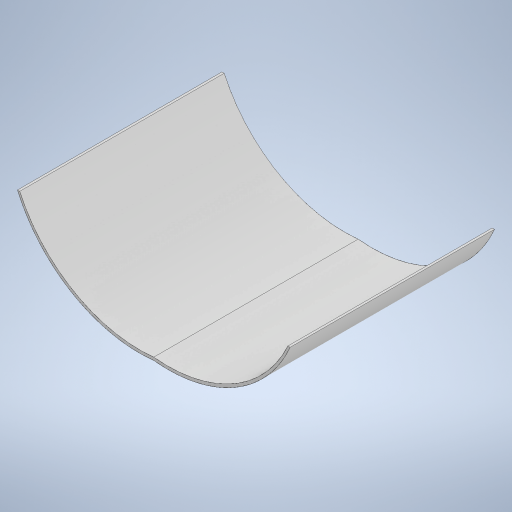
# Autodesk Inventor part: Base
Saved by Autodesk Inventor 2024 (Build 280153000, 153)
## iProperties
Created: 2024-09-04
Part Number: Base
Material: Generic
Document SubType Name: Modeling
Designer: srira
Density: 1 g/cm^3
Appearance: Default
Author: srira
Autodesk Inventor part; units mm, degrees
ref_plane "YZ Plane" through (0, 0, 0) normal (1, 0, 0) x (0, 1, 0)
ref_plane "XZ Plane" through (0, 0, 0) normal (0, 1, 0) x (-1, 0, 0)
ref_plane "XY Plane" through (0, 0, 0) normal (0, 0, 1) x (1, 0, 0)
sketch "Sketch1" plane through (0, 0, 0) normal (0, 0, 1) x (1, 0, 0)
  arc A0 (-600, 0) -> (0, -350.1196) centre (-63.3587, 230.4724) ccw
  arc A1 (-590, 0) -> (0, -337.4075) centre (-61.2566, 240.0264) ccw
  line L0 (0, -81.4327) -> (0, -44.5011)
  line L1 (-600, 0) -> (-590, 0)
  arc A2 (0, -350.1196) -> (600, 0) centre (63.3587, 230.4724) ccw
  arc A3 (0, -337.4075) -> (590, 0) centre (61.2566, 240.0264) ccw
  line L2 (600, 0) -> (590, 0)
  point P0 (0, 0)
  constraints: 8 point on circle, 6 end point, 4 centre point, 4 symmetric about line, 1 horizontal, 1 vertical, 2 other
extrude "Extrusion1" add sketch "Sketch1" along normal blind 900
body "Solid1"
